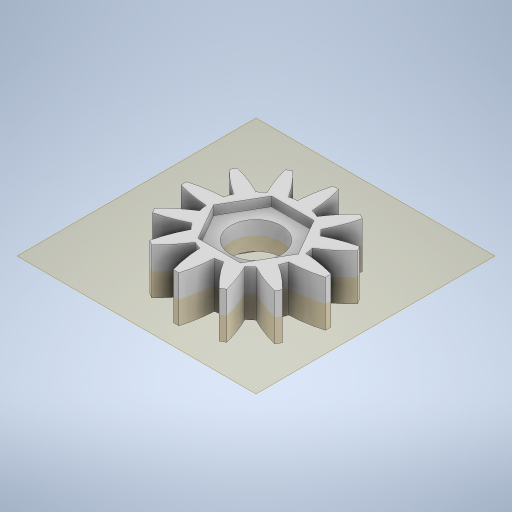
# Autodesk Inventor part: JointFixeSmallr
Saved by Autodesk Inventor 2023 (Build 270158000, 158)
## iProperties
Created: 2023-12-22
Part Number: JointFixeSmallr
Material: Generic
Document SubType Name: Modeling
Designer: Mustapha
Density: 1 g/cm^3
Appearance: Default
Author: Mustapha
Autodesk Inventor part; units mm, degrees
ref_plane "YZ Plane" through (0, 0, 0) normal (1, 0, 0) x (0, 1, 0)
ref_plane "XZ Plane" through (0, 0, 0) normal (0, 1, 0) x (-1, 0, 0)
ref_plane "XY Plane" through (0, 0, 0) normal (0, 0, 1) x (1, 0, 0)
sketch "Sketch1" plane through (0, 0, 0) normal (0, 1, 0) x (-1, 0, 0)
  circle A0 centre (0, 0) radius 5
  line L0 (5, 0) -> (9.8774, -1.3309) construction
  arc A1 (8.2733, -0.1123) -> (3.8334, 0.4702) centre (4.1778, -14.1163) ccw
  line L1 (9.8774, -1.3309) -> (5, 0) construction
  arc A2 (3.8334, -1.3043) -> (8.2733, -0.7218) centre (4.1778, 13.2822) ccw
  line L2 (3.8879, -2.2603) -> (3.8879, -0.5721)
  line L3 (3.8879, -0.262) -> (3.8879, 1.4262)
  line L4 (0.1623, -0.03) -> (0.1623, 0.0204)
  circle A3 centre (0, 0) radius 2.75
  line L5 (8.2733, -0.7218) -> (8.2733, -0.1123)
  arc A4 (3.972, 0.7871) -> (7.5258, 3.5116) centre (-3.023, 13.5916) ccw
  line L6 (7.5258, 3.5116) -> (7.2211, 4.0394)
  arc A5 (7.2211, 4.0394) -> (3.0847, 2.3239) centre (10.6762, -10.1362) ccw
  arc A6 (3.0463, 2.6677) -> (4.7618, 6.804) centre (-9.4138, 10.2592) ccw
  line L7 (4.7618, 6.804) -> (4.2339, 7.1088)
  arc A7 (4.2339, 7.1088) -> (1.5095, 3.5549) centre (14.314, -3.4401) ccw
  arc A8 (1.3043, 3.8334) -> (0.7218, 8.2733) centre (-13.2822, 4.1778) ccw
  line L8 (0.7218, 8.2733) -> (0.1123, 8.2733)
  arc A9 (0.1123, 8.2733) -> (-0.4702, 3.8334) centre (14.1163, 4.1778) ccw
  arc A10 (-0.7871, 3.972) -> (-3.5116, 7.5258) centre (-13.5916, -3.023) ccw
  line L9 (-3.5116, 7.5258) -> (-4.0394, 7.2211)
  arc A11 (-4.0394, 7.2211) -> (-2.3239, 3.0847) centre (10.1362, 10.6762) ccw
  arc A12 (-2.6677, 3.0463) -> (-6.804, 4.7618) centre (-10.2592, -9.4138) ccw
  line L10 (-6.804, 4.7618) -> (-7.1088, 4.2339)
  arc A13 (-7.1088, 4.2339) -> (-3.5549, 1.5095) centre (3.4401, 14.314) ccw
  arc A14 (-3.8334, 1.3043) -> (-8.2733, 0.7218) centre (-4.1778, -13.2822) ccw
  line L11 (-8.2733, 0.7218) -> (-8.2733, 0.1123)
  arc A15 (-8.2733, 0.1123) -> (-3.8334, -0.4702) centre (-4.1778, 14.1163) ccw
  arc A16 (-3.972, -0.7871) -> (-7.5258, -3.5116) centre (3.023, -13.5916) ccw
  line L12 (-7.5258, -3.5116) -> (-7.2211, -4.0394)
  arc A17 (-7.2211, -4.0394) -> (-3.0847, -2.3239) centre (-10.6762, 10.1362) ccw
  arc A18 (-3.0463, -2.6677) -> (-4.7618, -6.804) centre (9.4138, -10.2592) ccw
  line L13 (-4.7618, -6.804) -> (-4.2339, -7.1088)
  arc A19 (-4.2339, -7.1088) -> (-1.5095, -3.5549) centre (-14.314, 3.4401) ccw
  arc A20 (-1.3043, -3.8334) -> (-0.7218, -8.2733) centre (13.2822, -4.1778) ccw
  line L14 (-0.7218, -8.2733) -> (-0.1123, -8.2733)
  arc A21 (-0.1123, -8.2733) -> (0.4702, -3.8334) centre (-14.1163, -4.1778) ccw
  arc A22 (0.7871, -3.972) -> (3.5116, -7.5258) centre (13.5916, 3.023) ccw
  line L15 (3.5116, -7.5258) -> (4.0394, -7.2211)
  arc A23 (4.0394, -7.2211) -> (2.3239, -3.0847) centre (-10.1362, -10.6762) ccw
  arc A24 (2.6677, -3.0463) -> (6.804, -4.7618) centre (10.2592, 9.4138) ccw
  line L16 (6.804, -4.7618) -> (7.1088, -4.2339)
  arc A25 (7.1088, -4.2339) -> (3.5549, -1.5095) centre (-3.4401, -14.314) ccw
  point P0 (4.8297, -1.2938)
  point P1 (4.9795, 0.4523)
  point P2 (4.0863, 2.8814)
  point P3 (4.8296, 1.2944)
  point P4 (2.0981, 4.5385)
  point P5 (3.5353, 3.5357)
  point P6 (-0.4523, 4.9795)
  point P7 (1.2938, 4.8297)
  point P8 (-2.8814, 4.0863)
  point P9 (-1.2944, 4.8296)
  point P10 (-4.5385, 2.0981)
  point P11 (-3.5357, 3.5353)
  point P12 (-4.9795, -0.4523)
  point P13 (-4.8297, 1.2938)
  point P14 (-4.0863, -2.8814)
  point P15 (-4.8296, -1.2944)
  point P16 (-2.0981, -4.5385)
  point P17 (-3.5353, -3.5357)
  point P18 (0.4523, -4.9795)
  point P19 (-1.2938, -4.8297)
  point P20 (2.8814, -4.0863)
  point P21 (1.2944, -4.8296)
  point P22 (4.5385, -2.0981)
  point P23 (3.5357, -3.5353)
  dimension "d0" = 10
  dimension "d5" = 5.5
  dimension "d14" = 360
  constraints: 48 point on circle, 34 end point, 25 centre point, 2 coincident, 1 vertical, 111 other
  measures "d5" diameter of A3
extrude "Extrusion1" add sketch "Sketch1" along normal blind 5
sketch "Sketch2" plane through (0, 5, 0) normal (0, 1, 0) x (1, 0, 0)
  line L0 (-2.3094, 4) -> (2.3094, 4)
  line L1 (2.3094, 4) -> (4.6188, 0)
  line L2 (4.6188, 0) -> (2.3094, -4)
  line L3 (2.3094, -4) -> (-2.3094, -4)
  line L4 (-2.3094, -4) -> (-4.6188, 0)
  line L5 (-4.6188, 0) -> (-2.3094, 4)
  line L6 (0, 0) -> (-6.3613, 0)
  dimension "d8" = 8
  constraints: 14 end point, 1 coincident, 1 horizontal, 1 parallel, 13 other
  measures "d8" distance between parallel lines of L3 L0
extrude "Extrusion2" cut sketch "Sketch2" against normal blind 1
ref_plane "Work Plane1" through (0, 2.5, 0) normal (0, 1, 0) x (1, 0, 0)
mirror "Mirror1" about plane through (0, 2.5, 0) normal (0, 1, 0) of "Extrusion2"
body "Solid1"
